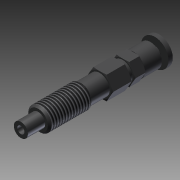
# Autodesk Inventor part: ZPT08U6-04_B_BUFFER
Saved by Autodesk Inventor 2011 SP1 (Build 150282100, 282)
## iProperties
Created: 2018-01-08
Part Number: ZPT08U6-04_B_BUFFER
Catalog Web Link: www.cadenas.de
Description: ZPT_2_8B_BUFFER-Vacuum Pad/Vertical Vacuum Entry With Buffer
Vendor: SMC
Document SubType Name: Modeling
Designer: psAdmin
Manufacturer: SMC
Mass: 1.8896 g
Surface Area: 17.6241 cm^2
Volume: 1.8896 cm^3
Density: 1 g/cm^3
Category: PARTsolutions
Company: SMC
Title: ZPT08U6-04_B_BUFFER
Author: Cadenas PARTsolutions
Comments: Vacuum Pad/Vertical Vacuum Entry With Buffer
PSOL_IDENT_0: {$CADENAS_DATA\23d-libs\smc_jp\vacuum_equipment\vacuum_pad\zp\zpt_b\zpt_2_8_b\parts\zpt_2_8_buffer_b
PSOL_IDENT_1: .prj},200 {VTYP=3D},{NB=ZPT08U6-04_B_BUFFER},{LINA=ZPT08U6-04_B_BUFFER},{NN=ZPT_2_8B_BUFFER},{DATE=1
PSOL_IDENT_2: 2.07.2017 07:16:19},{GEOMDATE=23.02.2011 00:59:00},{VERSION=},{LINEID=60},{LINESUBID=-1},{WBVAR=STRO
PSOL_IDENT_3: KE,PORT}  {NB=ZPT08U6-04_B_BUFFER},{LINA=ZPT08U6-04_B_BUFFER},{KT=DUMMY},{DIAMETER=8},{DIAMETERX=08}
PSOL_IDENT_4: ,{PAD=(U) Flat},{PADX=U},{STROKE=6},{PORT=04},{ORDER=ZPT08U6-04},{A=8.0},{B=9.0},{C=2.5},{Y=1.0},{D=
PSOL_IDENT_5: 18.0},{E=15.0},{G=44},{F=60},{DU=0.0},{EU=0.0}
NN: ZPT_2_8B_BUFFER
NT: Vacuum Pad/Vertical Vacuum Entry With Buffer
NB: ZPT08U6-04_B_BUFFER
NBSYN: $ORDER._B_BUFFER
LINA: ZPT08U6-04_B_BUFFER
DIAMETER: 8
PAD: (U) Flat
STROKE: 6
PORT: (04) dia 4 tube (One-touch fitting)
A: 8.0
B: 9.0
C: 2.5
Y: 1.0
D: 18.0
E: 15.0
DU: 0.0
EU: 0.0
SUPPLIER: SMC
ARTICLENO: ZPT08U6-04_B_BUFFER
BOMINFO: ZPT08U6-04_B_BUFFER
CREATOR: CADENAS GmbH
Autodesk Inventor part; units mm, degrees
sketch "Sketch_9" plane through (0, 0, 0) normal (0, 0, 1) x (1, 0, 0)
  line L0 (0, 12) -> (0, 60)
  line L1 (1.25, 60) -> (1.25, 12)
  line L2 (1.25, 12) -> (2.45, 12)
  line L3 (2.45, 12) -> (2.45, 18)
  line L4 (2.45, 18) -> (3.3865, 18)
  line L5 (3.3865, 18) -> (4, 18.6135)
  line L6 (4, 18.6135) -> (4, 32.3865)
  line L7 (4, 32.3865) -> (3.3865, 33)
  line L8 (3.3865, 33) -> (3.5, 33)
  line L9 (3.5, 33) -> (3.5, 39.35)
  line L10 (3.5, 39.35) -> (4, 39.35)
  line L11 (4, 39.35) -> (6.4, 39.9931)
  line L12 (6.4, 39.9931) -> (6.4, 45.3569)
  line L13 (6.4, 45.3569) -> (4, 46)
  line L14 (4, 46) -> (3.45, 46)
  line L15 (3.45, 46) -> (3.45, 47.3)
  line L16 (3.45, 47.3) -> (3.8105, 47.3)
  line L17 (3.8105, 47.3) -> (6.0968, 47.9126)
  line L18 (6.0968, 47.9126) -> (6.0968, 50.4874)
  line L19 (6.0968, 50.4874) -> (3.8105, 51.1)
  line L20 (3.8105, 51.1) -> (3.95, 51.1)
  line L21 (3.95, 51.1) -> (3.95, 57)
  line L22 (3.95, 57) -> (2.05, 57)
  line L23 (2.05, 57) -> (2.05, 58.5)
  line L24 (2.05, 58.5) -> (4.75, 58.5)
  line L25 (4.75, 58.5) -> (4.75, 60)
  line L26 (4.75, 60) -> (1.25, 60)
  constraints: 54 end point
revolve "Revolution1" add sketch "Sketch_9" angle 360 about axis through (0, 12, 0) along (0, -1, 0)
thread "Thread1" size "M8x1" class "6g" standard "ISO Metric profile" full length
sketch "Sketch_10" plane through (0, 51.1, 0) normal (0, 1, 0) x (1, 0, 0)
  circle A0 centre (0, 0) radius 8.8
  line L0 (-4.4, 0) -> (-2.2, -3.8105)
  line L1 (-2.2, -3.8105) -> (2.2, -3.8105)
  line L2 (2.2, -3.8105) -> (4.4, 0)
  line L3 (4.4, 0) -> (2.2, 3.8105)
  line L4 (2.2, 3.8105) -> (-2.2, 3.8105)
  line L5 (-2.2, 3.8105) -> (-4.4, 0)
  constraints: 12 end point, 1 centre point
extrude "Extrusion1" cut sketch "Sketch_10" against normal blind 3.8
sketch "Sketch_11" plane through (0, 46, 0) normal (0, 1, 0) x (1, 0, 0)
  circle A0 centre (0, 0) radius 8
  line L0 (-4.6188, 0) -> (-2.3094, -4)
  line L1 (-2.3094, -4) -> (2.3094, -4)
  line L2 (2.3094, -4) -> (4.6188, 0)
  line L3 (4.6188, 0) -> (2.3094, 4)
  line L4 (2.3094, 4) -> (-2.3094, 4)
  line L5 (-2.3094, 4) -> (-4.6188, 0)
  constraints: 12 end point, 1 centre point
extrude "Extrusion2" cut sketch "Sketch_11" against normal blind 6.65
ref_plane "BUFFER_DUMMY_XY" through (0, 0, 0) normal (0, -1, 0) x (1, 0, 0)
ref_plane "BUFFER_DUMMY_YZ" through (0, 0, 0) normal (1, 0, 0) x (0, 0, 1)
ref_plane "BUFFER_DUMMY_ZX" through (0, 0, 0) normal (0, 0, 1) x (0, -1, 0)
ref_plane "BUFFER_NUT1_XY" through (0, 25.5, 0) normal (0, 1, 0) x (1, 0, 0)
ref_plane "BUFFER_NUT1_YZ" through (0, 25.5, 0) normal (1, 0, 0) x (0, 0, -1)
ref_plane "BUFFER_NUT1_ZX" through (0, 25.5, 0) normal (0, 0, -1) x (0, 1, 0)
ref_plane "BUFFER_NUT2_XY" through (0, 25.5, 0) normal (0, 1, 0) x (1, 0, 0)
ref_plane "BUFFER_NUT2_YZ" through (0, 25.5, 0) normal (1, 0, 0) x (0, 0, -1)
ref_plane "BUFFER_NUT2_ZX" through (0, 25.5, 0) normal (0, 0, -1) x (0, 1, 0)
ref_plane "BUFFER_PLATE_XY" through (0, 25.5, 0) normal (0, 1, 0) x (1, 0, 0)
ref_plane "BUFFER_PLATE_YZ" through (0, 25.5, 0) normal (1, 0, 0) x (0, 0, -1)
ref_plane "BUFFER_PLATE_ZX" through (0, 25.5, 0) normal (0, 0, -1) x (0, 1, 0)
body "Solid1"
